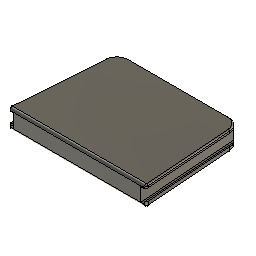
ID.3 Separator (Autodesk Fusion 360 design; units mm, degrees)
part number: 2026-04-10-16-56-54-716
Autodesk Fusion 360 part; units mm, degrees
note: some values were not read from the file. Set by a fixed rule: which sketch regions a step uses.
sketch "Sketch1" plane through (0, 0, 0) normal (0, 0, 1) x (1, 0, 0)
  line L0 (0, 0) -> (0.0278, 83.3)
  line L1 (0.0278, 83.3) -> (40.7389, 83.2864)
  line L2 (50.7086, 74.0194) -> (56.15, -0.0187)
  line L3 (56.15, -0.0187) -> (0, 0)
  line L4 (-50.6592, 74.0532) -> (-56.15, 0.0187)
  line L5 (0, 0) -> (0.0278, 83.3)
  line L6 (0.0278, 83.3) -> (-40.6833, 83.3136)
  line L7 (-56.15, 0.0187) -> (0, 0)
  arc A0 (50.7086, 74.0194) -> (40.7389, 83.2864) centre (40.7355, 73.2864) ccw
  arc A1 (-40.6833, 83.3136) -> (-50.6592, 74.0532) centre (-40.6866, 73.3136) ccw
  point P0 (50.0278, 83.2833)
  dimension "d4" = 56.15
  dimension "d5" = 50
  dimension "d6" = 83.3
  dimension "d9" = 10
  dimension "d10" = 10
  constraint coincident L0.start L3.end
  constraint perpendicular L0 L1
  constraint perpendicular L0 L3
  constraint symmetric L3.end L0 L5.start
  constraint symmetric L1.start L0 L5.end
  constraint symmetric L0 L2.end L4.end
  constraint symmetric L0 L3.end L5.start
  constraint coincident P0 L1
  constraint coincident P0 L2
  constraint tangent L1 A0
  constraint tangent L2 A0
  constraint tangent L4 A1
  constraint tangent L6 A1
  measures "d4" horizontal distance of L2.end L0.start
  measures "d5" horizontal distance of L0.end P0
  measures "d6" vertical distance of L0.start L0.end
  measures "d9" radius of A0
  measures "d10" radius of A1
extrude "Extrude1" add sketch "Sketch1" along normal blind 15.7
sketch "Sketch2" plane through (55.847, 4.1044, 0) normal (0.99731, 0.073296, 0) x (-0.073296, 0.99731, 0)
  line L0 (-4.1343, 0) -> (70.1035, 0)
  line L1 (70.1035, 0) -> (70.1035, 15.7)
  line L2 (70.1035, 15.7) -> (-4.1343, 15.7)
  line L3 (-4.1343, 15.7) -> (-4.1343, 0)
  line L4 (-4.1343, 13.2) -> (85.8724, 13.2)
  line L5 (85.8724, 13.2) -> (85.8724, 3.7)
  line L6 (85.8724, 3.7) -> (-4.1343, 3.7)
  line L7 (-4.1343, 3.7) -> (-4.1343, 13.2)
  dimension "d13" = 2.5
  dimension "d14" = 3.7
  constraint horizontal L4
  constraint vertical L5
  constraint horizontal L6
  constraint vertical L7
  constraint coincident L3 L4.start
  measures "d13" distance of L2 L4
  measures "d14" distance of L0 L6
sketch "Sketch4" plane through (-55.8442, 4.1417, 0) normal (-0.997261, 0.073962, 0) x (-0.073962, -0.997261, 0)
  line L0 (-70.1035, 0) -> (4.1343, 0)
  line L1 (4.1343, 0) -> (4.1343, 15.7)
  line L2 (4.1343, 15.7) -> (-70.1035, 15.7)
  line L3 (-70.1035, 15.7) -> (-70.1035, 0)
  line L4 (4.1343, 13.2) -> (-93, 13.2)
  line L5 (-93, 13.2) -> (-93, 3.7)
  line L6 (-93, 3.7) -> (4.1343, 3.7)
  line L7 (4.1343, 3.7) -> (4.1343, 13.2)
  dimension "d17" = 2.5
  dimension "d18" = 3.7
  constraint horizontal L4
  constraint vertical L5
  constraint horizontal L6
  constraint vertical L7
  constraint coincident L1 L4.start
  measures "d17" distance of L2 L4
  measures "d18" distance of L0 L6
extrude "Extrude2" cut sketch "Sketch4" against normal blind 4 contours L3 L4 L5 L6 | L1 L3 L4 L6 L7
extrude "Extrude3" cut sketch "Sketch2" against normal blind 4 contours L1 L3 L4 L6 L7 | L1 L4 L5 L6
sketch "Sketch8" plane through (0, 0, 3.7) normal (0, 0, 1) x (-1, 0, 0)
  line L0 (-52.1391, 0.0174) -> (-56.15, 0.0187)
  line L1 (-56.15, 0.0187) -> (-50.7086, -74.0194)
  line L2 (-46.133, -81.7047) -> (-52.1391, 0.0174)
  line L3 (-52.1391, 0.0174) -> (-54.9543, 0.0183)
  line L4 (-48.933, -81.9105) -> (-46.133, -81.7047)
  line L5 (-46.133, -81.7047) -> (-52.1391, 0.0174)
  line L6 (-48.933, -81.9105) -> (-54.9543, 0.0183)
  line L7 (0, -88) -> (0, 10)
  line L8 (48.933, -81.9105) -> (54.9543, 0.0183)
  line L9 (48.933, -81.9105) -> (46.133, -81.7047)
  line L10 (46.133, -81.7047) -> (52.1391, 0.0174)
  line L11 (52.1391, 0.0174) -> (54.9543, 0.0183)
  arc A0 (-50.7086, -74.0194) -> (-46.133, -81.7047) centre (-40.7355, -73.2864) ccw
  dimension "d27" = 2.8
  constraint coincident L0.start L2.end
  constraint coincident L0 L3.end
  constraint coincident L2.start L4.end
  constraint vertical L7
  constraint parallel L5 L6
  constraint symmetric L0.start L7 L10.end
  constraint symmetric L3.end L7 L8.end
  constraint symmetric L4.start L7 L8.start
  constraint symmetric L2.start L7 L9.end
  measures "d27" horizontal distance of L4.start L2.start
extrude "Extrude4" cut sketch "Sketch8" against normal blind 1.5 contours L0 L2 L3 L5 L6 A0 | L8 L9 L10 L11
fillet "Fillet1" radius 2 6 edges at (0, 0, 0) (0, 0, 15.7) (56.15, -0.0187, 14.45) (56.15, -0.0187, 1.85) (-56.15, 0.0187, 1.85) (-56.15, 0.0187, 14.45)
fillet "Fillet2" radius 1 9 edges at (55.4113, 0.5673, 15.1142) (55.9962, 2.055, 15.7) (53.3504, 38.074, 15.7) (47.5438, 80.6109, 15.7) (0.0278, 83.3, 15.7) (-47.4899, 80.6426, 15.7) (-53.325, 38.1096, 15.7) (-55.9948, 2.0924, 15.7) (-55.4109, 0.6043, 15.1142)
fillet "Fillet3" radius 1 9 edges at (-55.4109, 0.6043, 0.5858) (-55.9948, 2.0924, 0) (-53.325, 38.1096, 0) (-47.4899, 80.6426, 0) (0.0278, 83.3, 0) (47.5438, 80.6109, 0) (53.3504, 38.074, 0) (55.9962, 2.055, 0) (55.4113, 0.5673, 0.5858)
equation "d4 = ( 112.3 / 2 ) * 1 mm"
equation "d5 = ( 100 / 2 ) * 1 mm"
